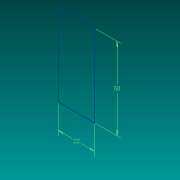
# Autodesk Inventor part: 连接块
Saved by Autodesk Inventor 2021 (Build 250183000, 183)
## iProperties
Created: 2025-04-18
Part Number: 连接块
Material: 常规
Document SubType Name: Modeling
Designer: 86155
Density: 1 g/cm^3
Appearance: 默认
Author: 86155
Autodesk Inventor part; units mm, degrees
ref_plane "YZ Plane" through (0, 0, 0) normal (1, 0, 0) x (0, 1, 0)
ref_plane "XZ Plane" through (0, 0, 0) normal (0, 1, 0) x (-1, 0, 0)
ref_plane "XY Plane" through (0, 0, 0) normal (0, 0, 1) x (1, 0, 0)
sketch "草图1" plane through (0, 0, 0) normal (0, 0, 1) x (1, 0, 0)
  line L0 (0, 0) -> (27, 0)
  line L1 (27, 0) -> (27, -45)
  line L2 (27, -45) -> (0, -45)
  line L3 (0, -45) -> (0, 0)
  dimension "d0" = 27
  dimension "d1" = 45
  constraints: 8 end point, 2 parallel, 1 horizontal, 1 perpendicular
  measures "d0" distance of L1.end L2.end
  measures "d1" distance of L0.end L1.end
extrude "拉伸1" add sketch "草图1" along normal blind 10
sketch "草图2" plane through (0, 0, 0) normal (0, 1, 0) x (1, 0, 0)
  circle A0 centre (32, -5) radius 5
  line L0 (27, -10) -> (0, -10) projected
  line L1 (27, 0) -> (27, -10) projected
  line L2 (0, 0) -> (27, 0) projected
  line L3 (32, 0) -> (27, 0)
  line L4 (27, 0) -> (27, -10) projected
  line L5 (27, -5) -> (27, 0)
  dimension "d4" = 10
  dimension "d5" = 5
  dimension "d6" = 5
  constraints: 4 end point, 1 collinear, 1 horizontal, 1 midpoint, 3 other
  measures "d5" distance from line of L0 point (32, -5)
  measures "d6" distance from line of L1 point (32, -5)
extrude "拉伸2" add sketch "草图2" against normal blind 15
sketch "草图3" plane through (0, 0, 10) normal (0, 1, 0) x (1, 0, 0)
  arc A0 (27, 5) -> (32, 10) centre (32, 5) ccw projected
  circle A1 centre (32, 5) radius 2.5
  point P0 (0, 10)
  dimension "d9" = 5
  constraints: 1 centre point, 1 coincident
  measures "d9" diameter of A1
ref_plane "工作平面1" through (0, -22.5, 0) normal (0, -1, 0) x (1, 0, 0)
mirror "镜像1" about plane through (0, -22.5, 0) normal (0, -1, 0) of "拉伸2"
extrude "拉伸3" cut sketch "草图3" against normal up to surface (45 mm away)
sketch "草图4" plane through (0, 0, 10) normal (0, 0, 1) x (1, 0, 0)
  line L0 (27, 0) -> (0, 0) projected
  line L1 (0, -45) -> (27, -45) projected
  line L2 (0, 0) -> (0, -45) projected
  point P0 (10, -12)
  point P1 (10, -33)
  dimension "d12" = 12
  dimension "d13" = 12
  dimension "d14" = 10
  dimension "d15" = 10
  measures "d12" distance from line of L0 point (10, -12)
  measures "d13" distance from line of L1 point (10, -33)
  measures "d14" distance from line of L2 point (10, -12)
  measures "d15" distance from line of L2 point (10, -33)
hole "孔1" at (10, -12, 10) at (10, -33, 10) direction (0, 0, -1) diameter 8.376 depth 27.3 thread size "M10x1.5" designation "M10" class "6H" standard "GB Metric profile"
